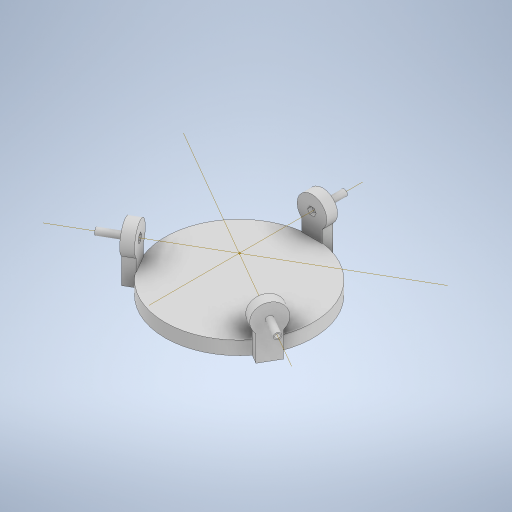
# Autodesk Inventor part: mobile_platform
Saved by Autodesk Inventor 2024 (Build 280153000, 153)
## iProperties
Created: 2023-10-31
Part Number: mobile_platform
Material: Generic
Document SubType Name: Modeling
Designer: MATEO
Density: 1 g/cm^3
Appearance: Default
Mass: 110.089 g
Surface Area: 292.867 cm^2
Volume: 110.089 cm^3
Author: MATEO
Autodesk Inventor part; units mm, degrees
ref_plane "YZ Plane" through (0, 0, 0) normal (1, 0, 0) x (0, 1, 0)
ref_plane "XZ Plane" through (0, 0, 0) normal (0, 1, 0) x (-1, 0, 0)
ref_plane "XY Plane" through (0, 0, 0) normal (0, 0, 1) x (1, 0, 0)
sketch "Sketch1" plane through (0, 0, 0) normal (0, 1, 0) x (-1, 0, 0)
  circle A0 centre (0, 0) radius 55
  dimension "d0" = 110
  constraints: 1 centre point, 1 coincident
  measures "d0" diameter of A0
extrude "Extrusion1" add sketch "Sketch1" against normal blind 10
sketch "Sketch2" plane through (0, 0, 0) normal (0, 1, 0) x (1, 0, 0)
  circle A0 centre (0, 0) radius 55 projected
  line L0 (-7.5, 54) -> (7.5, 54)
  line L1 (7.5, 54) -> (7.5, 62.0467)
  line L2 (7.5, 62.0467) -> (-7.5, 62.0467)
  line L3 (-7.5, 62.0467) -> (-7.5, 54)
  point P0 (0, 54)
  point P1 (7.5, 54.4862)
  point P2 (-7.5, 54.4862)
  point P3 (0, 62.0467)
  dimension "d3" = 15
  dimension "d4" = 8.0467
  dimension "d21" = 62.0467
  constraints: 8 end point, 2 midpoint, 2 parallel, 1 horizontal, 1 perpendicular, 1 vertical alignment
  measures "d3" distance of L2.end L1.end
  measures "d4" distance of L1.end L0.end
  measures "d21" distance of point (0, 0) point (0, 62.047)
extrude "Extrusion2" add sketch "Sketch2" along normal blind 5 and the other way blind 10 contours L1 L0 L3 A0 | A0 L3 L2 L1 picked at (0.8356, 54.3143)
sketch "Sketch3" plane through (-7.5, 0, -54) normal (0, 0, 1) x (1, 0, 0)
  line L0 (15, 0) -> (0, 0) projected
  line L1 (0, 5) -> (15, 5)
  line L2 (0, 5) -> (15, 5)
  line L3 (0, 5) -> (0, 8.9533)
  line L4 (15, 5) -> (15, 8.9533)
  arc A0 (15, 8.9533) -> (0, 8.9533) centre (7.5, 17) ccw
  line L5 (0, 5) -> (15, 5) projected
  point P0 (7.5, 0)
  point P1 (7.5, 0)
  point P2 (7.5, 5)
  point P3 (7.5, 5)
  dimension "d27" = 22
  dimension "d28" = 12
  dimension "d29" = 15
  constraints: 8 end point, 4 midpoint, 2 coincident, 2 horizontal alignment, 2 point on circle, 2 vertical, 1 centre point, 1 collinear, 1 vertical alignment
  measures "d27" diameter of A0
  measures "d28" distance from line of L1 A0.centre
  measures "d29" distance of L1.start L1.end
extrude "Extrusion3" add sketch "Sketch3" against normal up to surface (8.0467 mm away)
pattern_circular "Circular Pattern1" count 3 over 360 about axis through (0, 0, 0) along (0, -1, 0) of "Extrusion2", "Extrusion3"
sketch "Sketch5" plane through (-7.5, 0, -54) normal (0, 0, 1) x (1, 0, 0)
  arc A0 (15, 8.9533) -> (0, 8.9533) centre (7.5, 17) ccw projected
  circle A1 centre (7.5, 17) radius 2.4
  point P0 (7.5, 0)
  dimension "d30" = 4.8
  constraints: 1 centre point, 1 coincident
  measures "d30" diameter of A1
extrude "Extrusion5" add sketch "Sketch5" against normal blind 24
pattern_circular "Circular Pattern3" count 3 over 360 about axis through (0, 0, 0) along (0, -1, 0) of "Extrusion5"
sketch "Sketch6" plane through (-50.5154, 0, 20.5048) normal (0.866, 0, -0.5) x (-0.5, 0, -0.866)
  arc A0 (0, 8.9533) -> (-15, 8.9533) centre (-7.5, 17) ccw projected
  arc A1 (0, 8.9533) -> (-15, 8.9533) centre (-7.5, 17) ccw projected
  line L0 (-4.3246, 17) -> (-5.9123, 14.25)
  line L1 (-5.9123, 14.25) -> (-9.0877, 14.25)
  line L2 (-9.0877, 14.25) -> (-10.6754, 17)
  line L3 (-10.6754, 17) -> (-9.0877, 19.75)
  line L4 (-9.0877, 19.75) -> (-5.9123, 19.75)
  line L5 (-5.9123, 19.75) -> (-4.3246, 17)
  point P0 (-7.5, 0)
  dimension "d36" = 5.5
  constraints: 12 end point, 2 coincident, 1 horizontal alignment, 13 other
  measures "d36" distance between parallel lines of L1 L4
extrude "Extrusion6" cut sketch "Sketch6" against normal blind 3
sketch "Sketch7" plane through (-53.1134, 0, 22.0048) normal (0.866, 0, -0.5) x (-0.5, 0, -0.866)
  circle A0 centre (-7.5, 17) radius 1.6
  line L0 (-9.0877, 19.75) -> (-5.9123, 19.75) projected
  line L1 (-10.6754, 17) -> (-9.0877, 19.75) projected
  line L2 (-9.0877, 14.25) -> (-10.6754, 17) projected
  line L3 (-5.9123, 14.25) -> (-9.0877, 14.25) projected
  line L4 (-4.3246, 17) -> (-5.9123, 14.25) projected
  line L5 (-5.9123, 19.75) -> (-4.3246, 17) projected
  point P0 (-7.5, 0)
  point P1 (-7.5, 14.25)
  dimension "d39" = 3.2
  constraints: 1 centre point, 1 horizontal alignment, 1 midpoint, 1 vertical alignment
  measures "d39" diameter of A0
extrude "Extrusion7" cut sketch "Sketch7" against normal through all contours A0
pattern_circular "Circular Pattern4" count 3 over 360 about axis through (0, 0, 0) along (0, -1, 0) of "Extrusion6", "Extrusion7"
body "Solid1"
